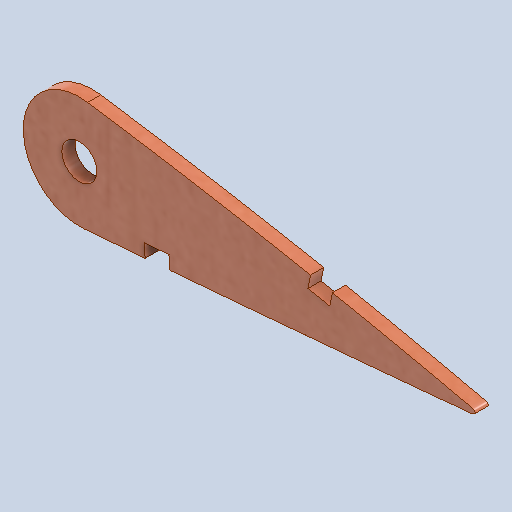
# Autodesk Inventor part: 2P.03.01.10.IM.AileronRibEnd
Saved by Autodesk Inventor 2025.2 (Build 292293000, 293)
## iProperties
Created: 2025-01-05
Part Number: 2P.03.01.10.IM.AileronRibEnd
Material: Wood (Walnut)
Document SubType Name: Modeling
Designer: Imist
Density: 0.55 g/cm^3
Appearance: Walnut - Natural Polished
Author: Imist
Autodesk Inventor part; units mm, degrees
ref_plane "YZ Plane" through (0, 0, 0) normal (1, 0, 0) x (0, 1, 0)
ref_plane "XZ Plane" through (0, 0, 0) normal (0, 1, 0) x (-1, 0, 0)
ref_plane "XY Plane" through (0, 0, 0) normal (0, 0, 1) x (1, 0, 0)
sketch "Sketch1" plane through (0, 0, 0) normal (0, 0, 1) x (1, 0, 0)
  line L0 (13.1712, 7.8143) -> (13.7511, 10.7577)
  line L1 (18.1712, 6.8292) -> (13.1712, 7.8143)
  line L2 (18.7511, 9.7726) -> (18.1712, 6.8292)
  line L3 (13.7511, 10.7577) -> (18.7511, 9.7726)
  spline S0 degree 4 poles (-37.1283, 19.4565) (-31.988, 18.6863) (-23.4121, 17.3807) (-12.0911, 15.51) (1.6086, 13.0716) (12.5956, 11.0074) (22.3539, 9.0584) (30.8015, 7.3391) (37.7818, 5.7744) (44.5921, 4.402) (48.6091, 3.1954) (51.1274, 3.1295) (51.4317, 2.2875) knots 0 0 0 0 0 0.183688 0.302378 0.416104 0.523956 0.624947 0.717922 0.80148 0.87369 1 1 1 1 1
  spline S1 degree 2 poles (-25.5579, 11.4472) (-25.4492, 11.4311) (-25.3406, 11.415) knots 0 0 0 1 1 1
  line L4 (-25.3627, 11.4183) -> (-25.3184, 11.4117) construction
  arc A0 (-25.3228, 11.4123) -> (-25.3583, 11.4176) centre (-40.9202, -93.4089) ccw construction
  line L5 (-18.3314, -4.3384) -> (-18.579, -1.3486)
  line L6 (-18.579, -1.3486) -> (-24.2449, -1.8177)
  line L7 (-24.2449, -1.8177) -> (-23.9973, -4.8075)
  line L8 (-23.9973, -4.8075) -> (-18.3314, -4.3384)
  arc A1 (-37.1283, 19.4565) -> (-37.9863, -5.9475) centre (-39.024, 6.804) ccw
  circle A2 centre (-39.024, 6.804) radius 4
  arc A3 (-4.8976, -3.2036) -> (-5.6763, -3.2701) centre (-4.5845, -11.4705) ccw
  line L9 (-20.3196, -4.5041) -> (-16.3432, -4.1726) construction
  arc A4 (-16.7409, -4.2059) -> (-19.922, -4.4711) centre (806.8876, -9970.2309) ccw construction
  spline S2 degree 4 poles (-37.9863, -5.9475) (-32.2632, -5.4818) (-24.0283, -4.8136) (-21.9434, -4.6394) (-18.3314, -4.3384) knots 0 0 0 0 0 1 1 1 1 1
  line L10 (-4.9769, -3.2104) -> (-4.8183, -3.1968) construction
  arc A5 (-4.9611, -3.209) -> (-4.8341, -3.1982) centre (-409.3906, 4736.1469) ccw construction
  spline S3 degree 2 poles (-5.6763, -3.2701) (-5.2865, -3.2368) (-4.8976, -3.2036) knots 0 0 0 1 1 1
  spline S4 degree 4 poles (12.0721, -1.7407) (12.5689, -1.6971) (12.7415, -1.6826) (25.5782, -0.5454) (30.0305, -0.1541) (37.6648, 0.5922) (44.2904, 1.0787) (48.5486, 1.7611) (51.0075, 1.4976) (51.4317, 2.2875) knots 0 0 0 0 0 0.172623 0.316544 0.485874 0.63811 0.76971 1 1 1 1 1
  line L11 (7.463, -2.1449) -> (16.6812, -1.3365) construction
  arc A6 (15.7599, -1.4238) -> (8.3854, -2.0706) centre (103.7869, -1047.5009) ccw construction
  line L12 (-18.3314, -4.3384) -> (-10.8115, -3.7157) construction
  line L13 (-10.8115, -3.7157) -> (1.428, -2.7022) construction
  line L14 (1.428, -2.7022) -> (12.5757, -1.6965) construction
  spline S5 degree 3 poles (-18.3314, -4.3384) (-10.8115, -3.7157) (1.428, -2.7022) (12.5757, -1.6965) knots 1 1 1 1 2 2 2 2
  point P0 (0, 0)
  point P1 (15.4403, -7.1521)
  point P2 (-2.5033, 3.2923)
  point P3 (-23.1393, 17.2995)
  point P4 (-9.9873, 15.1095)
  point P5 (2.1777, 12.9435)
  point P6 (13.2327, 10.8585)
  point P7 (23.0577, 8.9085)
  point P8 (31.5477, 7.1475)
  point P9 (38.6187, 5.6235)
  point P10 (44.1927, 4.3875)
  point P11 (48.2187, 3.4755)
  point P12 (50.6487, 2.9175)
  point P13 (-10.8115, -3.7157)
  point P14 (1.428, -2.7022)
  point P15 (31.1217, -0.0405)
  point P16 (38.3097, 0.6165)
  point P17 (43.9857, 1.1445)
  point P18 (48.0897, 1.5315)
  point P19 (50.5707, 1.7685)
  point P20 (-51.8103, 7.2396)
  point P21 (51.4317, 2.7285)
  point P22 (-51.8103, 21.5235)
  point P23 (-52.6203, -7.1085)
  point P24 (51.4317, 1.8465)
  point P25 (-37.1283, 6.7894)
  point P26 (-23.1393, 6.2818)
  point P27 (-9.9873, 5.7367)
  point P28 (2.1777, 5.1731)
  point P29 (13.2327, 4.61)
  point P30 (23.0577, 4.0701)
  point P31 (31.5477, 3.573)
  point P32 (38.6187, 3.1344)
  point P33 (44.1927, 2.7757)
  point P34 (48.2187, 2.5096)
  point P35 (50.6487, 2.3465)
  point P36 (-25.9011, 1.2856)
  point P37 (9.8661, 4.5796)
  point P38 (-19.9623, 10.5844)
  point P39 (-14.7015, 9.7084)
  point P40 (-9.8355, 8.842)
  point P41 (-5.4135, 8.008)
  point P42 (-1.4835, 7.228)
  point P43 (1.9125, 6.5236)
  point P44 (4.7409, 5.914)
  point P45 (6.9705, 5.4196)
  point P46 (8.5809, 5.0548)
  point P47 (9.5529, 4.8316)
  point P48 (-20.3055, 1.7416)
  point P49 (-15.0315, 2.182)
  point P50 (-10.1367, 2.5996)
  point P51 (-5.6763, 2.986)
  point P52 (-1.7019, 3.3376)
  point P53 (1.7421, 3.6484)
  point P54 (4.6173, 3.9112)
  point P55 (6.8877, 4.1224)
  point P56 (8.5293, 4.2772)
  point P57 (9.5217, 4.372)
  point P58 (12.0721, -1.7407)
  dimension "d0" = 3
  dimension "d1" = 5
  dimension "d2" = 52.7751
  dimension "d3" = 3
  dimension "d4" = 5.6658
  dimension "d5" = 8
  constraints: 24 end point, 9 point on circle, 8 midpoint, 7 centre point, 4 parallel, 3 coincident, 2 perpendicular, 1 point on line, 1 tangent, 43 other
  measures "d0" distance of L3.end L1.start
  measures "d1" horizontal distance of L3.end L0.end
  measures "d2" horizontal distance of A1.centre L0.end
  measures "d3" distance of L5.end L5.start
  measures "d4" horizontal distance of L5.end L6.end
  measures "d5" diameter of A2
extrude "Extrusion1" add sketch "Sketch1" along normal blind 3 contours L1 L2 S0 S4 S5 L5 L6 L7 S2 A1 L0
body "Solid1"
